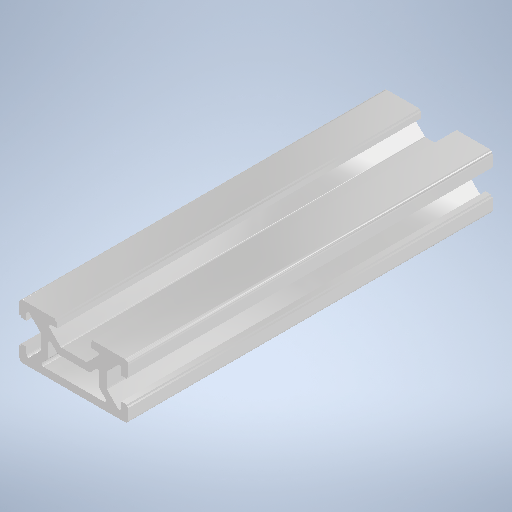
# Autodesk Inventor part: 15mm
Saved by Autodesk Inventor 2025.2 (Build 292293000, 293)
## iProperties
Created: 2025-04-03
Part Number: 15mm
Material: Aluminum 6061
Document SubType Name: Modeling
Designer: ishad
Density: 2.7 g/cm^3
Appearance: Aluminum - Polished
Author: ishad
Autodesk Inventor part; units mm, degrees
ref_plane "YZ Plane" through (0, 0, 0) normal (1, 0, 0) x (0, 1, 0)
ref_plane "XZ Plane" through (0, 0, 0) normal (0, 1, 0) x (-1, 0, 0)
ref_plane "XY Plane" through (0, 0, 0) normal (0, 0, 1) x (1, 0, 0)
sketch "Sketch1" plane through (0, 0, 0) normal (0, 0, 1) x (1, 0, 0)
  line L0 (-15, 0) -> (-15, 15) construction
  line L1 (-15, 15) -> (-4.5716, 15) construction
  line L2 (-15, 10.6) -> (-15, 4.4) construction
  line L3 (-15, 10.6) -> (-14.5, 10.6) construction
  line L4 (-14.5, 10.6) -> (-14.5, 11.1)
  line L5 (-14.5, 11.1) -> (-15, 11.1)
  line L6 (-15, 11.1) -> (-15, 10.6) construction
  line L7 (-14.5, 10.6) -> (-13, 10.6)
  line L8 (-15, 15) -> (-15, 11.1)
  line L9 (-13, 13.6) -> (-13, 10.6)
  line L10 (-13, 13.6) -> (-9, 9.6)
  line L11 (-9, 9.6) -> (-9, 7.5)
  line L12 (-15, 7.5) -> (0, 7.5) construction
  line L13 (-9, 7.5) -> (-9, 5.4)
  line L14 (-9, 5.4) -> (-13, 1.4)
  line L15 (-13, 4.4) -> (-13, 1.4)
  line L16 (-15, 4.4) -> (-14.5, 4.4) construction
  line L17 (-14.5, 4.4) -> (-14.5, 3.9)
  line L18 (-14.5, 3.9) -> (-15, 3.9)
  line L19 (-15, 3.9) -> (-15, 4.4) construction
  line L20 (-14.5, 4.4) -> (-13, 4.4)
  line L21 (-4.5716, 15) -> (-5.0716, 15) construction
  line L22 (-5.0716, 15) -> (-5.0716, 14.5)
  line L23 (-5.0716, 14.5) -> (-4.5716, 14.5)
  line L24 (-4.5716, 14.5) -> (-4.5716, 15) construction
  line L25 (-4.5716, 14.5) -> (-4.5716, 13)
  line L26 (-4.5716, 13) -> (-7.5716, 13)
  line L27 (-7.5716, 13) -> (-3.5716, 9)
  line L28 (-3.5716, 9) -> (0, 9)
  line L29 (-15, 3.9) -> (-15, 0)
  line L30 (-15, 0) -> (0, 0)
  line L31 (-4.4, 7) -> (0, 7)
  line L32 (-7, 9.6) -> (-4.4, 7)
  line L33 (-7, 9.6) -> (-7, 4.5716)
  line L34 (-7, 4.5716) -> (-9.5716, 2)
  line L35 (-9.5716, 2) -> (0, 2)
  line L36 (0, 2) -> (0, 0)
  line L37 (0, 9) -> (0, 7)
  line L38 (-15, 15) -> (-5.0716, 15)
  point P0 (-15, 10.85)
  point P1 (-9, 6.45)
  point P2 (-9, 8.55)
  point P3 (-1.7858, 9)
  point P4 (-5.5716, 11)
  dimension "d78" = 15
  dimension "d87" = 6.2
  dimension "d89" = 15
  dimension "d91" = 0.5
  dimension "d92" = 2
  dimension "d93" = 6
  dimension "d96" = 45
  dimension "d97" = 3
  dimension "d98" = 45
  dimension "d121" = 2
  dimension "d122" = 2
  dimension "d124" = 2
  dimension "d126" = 2
  dimension "d127" = 2
  constraints: 78 end point, 12 horizontal, 12 vertical, 11 equal length, 8 parallel, 7 midpoint, 4 perpendicular, 4 vertical alignment, 3 coincident, 3 horizontal alignment, 2 other
  measures "d78" distance of point (0, 0) L0.start
  measures "d87" distance of L2.start L2.end
  measures "d89" horizontal distance of point (0, 0) L0.end
  measures "d91" distance of L4.end L5.end
  measures "d92" distance of L2.start L7.end
  measures "d93" distance from line of point (-15, 10.85) L11
  measures "d96" angle of L10 L9
  measures "d97" distance of L9.start L7.end
  measures "d98" angle of L26 L27
  measures "d121" distance between parallel lines of L31 L28
  measures "d122" distance between parallel lines of L27 L32
  measures "d124" distance between parallel lines of L14 L34
  measures "d126" distance between parallel lines of L13 L33
  measures "d127" distance between parallel lines of L30 L35
extrude "Extrusion1" add sketch "Sketch1" along normal mid plane 100
mirror "Mirror1" about plane through (0, 0, 0) normal (1, 0, 0) of "Extrusion1"
fillet "Fillet1" radius 1 4 edges at (-15, 15, 0) (15, 15, 0) (15, 0, 0) (-15, 0, 0)
fillet "Fillet2" radius 0.5 18 edges at (-13, 13.6, 0) (-9, 9.6, 0) (-9, 5.4, 0) (-13, 1.4, 0) (-7, 9.6, 0) (-7, 4.5716, 0) (-9.5716, 2, 0) (-3.5716, 9, 0) (9, 5.4, 0) (-7.5716, 13, 0) (3.5716, 9, 0) (9.5716, 2, 0) (7, 4.5716, 0) (7.5716, 13, 0) (13, 1.4, 0) (9, 9.6, 0) (13, 13.6, 0) (7, 9.6, 0)
equation "\"d98\" = d96"
body "Solid1"
